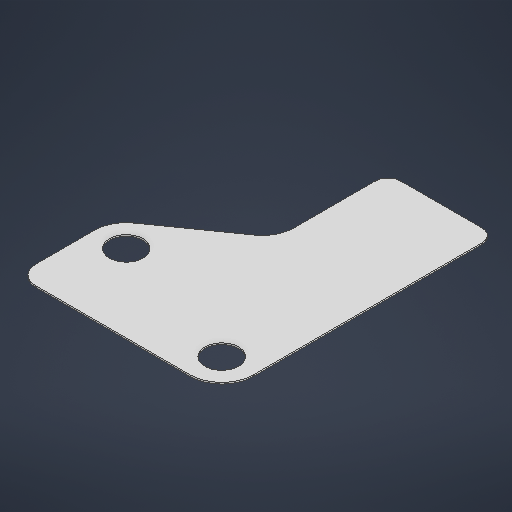
# Autodesk Inventor part: core_housing_master
Saved by Autodesk Inventor 2026 (Build 300175000, 175)
## iProperties
Created: 2025-05-09
Part Number: core_housing_master
Material: Generic
Document SubType Name: Modeling
Designer: Paul Juschitz
Density: 1 g/cm^3
Appearance: Default
d0: 1,000 ul
d1: 1,000 ul
d2: 151,500 mm
d3: 14,300 mm
d4: 5,000 ul
d8: 54,000 mm
d9: 5,000 mm
d10: 2,000 mm
core_housing_foot_outer_spacing: 10,000 mm
d12: 10,000 mm
core_housing_outset: 80,000 mm
d16: 10,000 mm
core_housing_foot_inner_spacing: 2,000 mm
d18: 2,000 mm
d19: 0,800 mm
d20: 0,00 deg
core_housing_tolerance: 0,200 mm
core_housing_material_thickness: 0,800 mm
d6: 360,00 deg
m2m_bottom_cover_diameter: 151,500 mm
m2m_bottom_foot_diameter: 14,300 mm
core_outer_width: 54,000 mm
core_outer_radius: 5,000 mm
core_height: 25,000 mm
core_inner_width: 50,400 mm
Author: Paul Juschitz
Autodesk Inventor part; units mm, degrees
ref_plane "YZ Plane" through (0, 0, 0) normal (1, 0, 0) x (0, 1, 0)
ref_plane "XZ Plane" through (0, 0, 0) normal (0, 1, 0) x (-1, 0, 0)
ref_plane "XY Plane" through (0, 0, 0) normal (0, 0, 1) x (1, 0, 0)
derived "m2m_bottom_2.ipt"
derived "core_dummy_1.ipt"
sketch "Sketch1" plane through (0, 0, 0) normal (0, 1, 0) x (-1, 0, 0)
  circle A0 centre (0, 0) radius 75.75 construction
  circle A1 centre (68.6, 0) radius 7.15 construction
  circle A2 centre (21.1986, 65.2425) radius 7.15 construction
  circle A3 centre (-55.4986, 40.3221) radius 7.15 construction
  circle A4 centre (-55.4986, -40.3221) radius 7.15 construction
  circle A5 centre (21.1986, -65.2425) radius 7.15 construction
  line L0 (-21.6486, -115.3221) -> (-65.6486, -115.3221) construction
  line L1 (-70.6486, -120.3221) -> (-70.6486, -164.3221) construction
  line L2 (-65.6486, -169.3221) -> (-21.6486, -169.3221) construction
  line L3 (-16.6486, -164.3221) -> (-16.6486, -120.3221) construction
  arc A6 (-16.6486, -120.3221) -> (-21.6486, -115.3221) centre (-21.6486, -120.3221) ccw construction
  arc A7 (-21.6486, -169.3221) -> (-16.6486, -164.3221) centre (-21.6486, -164.3221) ccw construction
  arc A8 (-70.6486, -164.3221) -> (-65.6486, -169.3221) centre (-65.6486, -164.3221) ccw construction
  arc A9 (-65.6486, -115.3221) -> (-70.6486, -120.3221) centre (-65.6486, -120.3221) ccw construction
  line L4 (-65.6486, -113.3221) -> (-21.6486, -113.3221) construction
  arc A10 (-14.6486, -120.3221) -> (-21.6486, -113.3221) centre (-21.6486, -120.3221) ccw construction
  line L5 (-14.6486, -120.3221) -> (-14.6486, -164.3221)
  arc A11 (-21.6486, -171.3221) -> (-14.6486, -164.3221) centre (-21.6486, -164.3221) ccw
  line L6 (-21.6486, -171.3221) -> (-65.6486, -171.3221)
  arc A12 (-72.6486, -164.3221) -> (-65.6486, -171.3221) centre (-65.6486, -164.3221) ccw
  line L7 (-72.6486, -164.3221) -> (-72.6486, -120.3221)
  arc A13 (-65.6486, -113.3221) -> (-72.6486, -120.3221) centre (-65.6486, -120.3221) ccw construction
  line L8 (-72.6486, -120.3221) -> (-72.6486, -40.3221)
  arc A14 (-55.4986, -23.1721) -> (-72.6486, -40.3221) centre (-55.4986, -40.3221) ccw
  line L9 (-55.4986, -23.1721) -> (28.3486, -23.1721)
  line L10 (38.3486, -33.1721) -> (38.3486, -65.2425)
  arc A15 (31.0636, -79.2711) -> (38.3486, -65.2425) centre (21.1986, -65.2425) ccw
  line L11 (31.0636, -79.2711) -> (-7.3636, -106.2934)
  arc A16 (-7.3636, -106.2934) -> (-14.6486, -120.3221) centre (2.5014, -120.3221) ccw
  arc A17 (38.3486, -33.1721) -> (28.3486, -23.1721) centre (28.3486, -33.1721) ccw
  circle A18 centre (21.1986, -65.2425) radius 9.15
  circle A19 centre (-55.4986, -40.3221) radius 9.15
  point P0 (-70.6486, -169.3221)
  point P1 (-70.6486, -115.3221)
  point P2 (38.3486, -23.1721)
  dimension "d2" = 151.5
  dimension "d3" = 14.3
  dimension "d6" = 360
  dimension "d8" = 54
  dimension "d9" = 5
  dimension "d10" = 2
  dimension "core_housing_foot_outer_spacing" = 10
  dimension "d12" = 10
  dimension "core_housing_outset" = 80
  dimension "d16" = 10
  dimension "core_housing_foot_inner_spacing" = 2
  dimension "d18" = 2
  constraints: 24 end point, 24 point on circle, 20 centre point, 17 tangent, 6 point on line, 5 perpendicular, 4 equal radius, 4 parallel, 2 concentric, 1 coincident, 1 horizontal, 1 horizontal alignment, 1 vertical, 18 other
  measures "d2" diameter of A0
  measures "d3" diameter of A1
  measures "d8" distance of point (-70.649, -115.322) point (-70.649, -169.322)
  measures "d9" radius of A6
  measures "d10" distance between parallel lines of L0 L4
  measures "core_housing_foot_outer_spacing" radial gap between concentric circles of A4 A14
  measures "d12" radial gap between concentric circles of A5 A15
  measures "core_housing_outset" distance of L7.end L8.end
  measures "d16" radius of A17
  measures "core_housing_foot_inner_spacing" radial gap between concentric circles of A5 A18
  measures "d18" radial gap between concentric circles of A4 A19
extrude "Extrusion2" add sketch "Sketch1" along normal blind 0.8
equation "\"d2\" = m2m_bottom_cover_diameter"
equation "\"d3\" = m2m_bottom_foot_diameter"
equation "\"d8\" = core_outer_width"
equation "\"d9\" = core_outer_radius"
equation "\"d10\" = 2 * core_housing_material_thickness + 2 * core_housing_tolerance"
equation "\"d12\" = core_housing_foot_outer_spacing"
equation "\"d16\" = core_housing_foot_outer_spacing"
equation "\"d18\" = core_housing_foot_inner_spacing"
equation "\"d19\" = core_housing_material_thickness"
equation "\"core_housing_tolerance\" = 0.2"
equation "\"core_housing_material_thickness\" = 0.8"
equation "\"m2m_bottom_cover_diameter\" = 151.5"
equation "\"m2m_bottom_foot_diameter\" = 14.3"
equation "\"core_outer_radius\" = 5"
equation "\"core_outer_width\" = 54"
body "Solid2"
